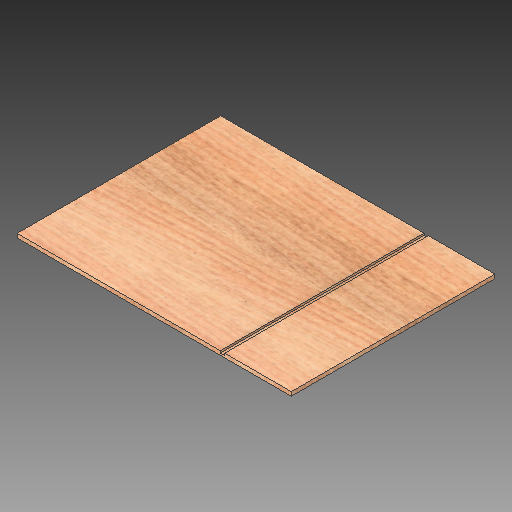
# Autodesk Inventor part: planche_bas
Saved by Autodesk Inventor 2019 (Build 230136000, 136)
## iProperties
Created: 2018-12-03
Part Number: planche_bas
Material: Wood (Birch)
Document SubType Name: Modeling
Designer: Bienvenue
Density: 0.55 g/cm^3
Appearance: Birch - Natural Polished
Author: Bienvenue
Autodesk Inventor part; units mm, degrees
ref_plane "YZ Plane" through (0, 0, 0) normal (1, 0, 0) x (0, 1, 0)
ref_plane "XZ Plane" through (0, 0, 0) normal (0, 1, 0) x (-1, 0, 0)
ref_plane "XY Plane" through (0, 0, 0) normal (0, 0, 1) x (1, 0, 0)
sketch "Sketch1" plane through (0, 0, 0) normal (0, 1, 0) x (-1, 0, 0)
  line L0 (0, 0) -> (412, 0)
  line L1 (412, 0) -> (412, -306)
  line L2 (412, -306) -> (0, -306)
  line L3 (0, -306) -> (0, 0)
  dimension "d0" = 306
  dimension "d1" = 412
  constraints: 8 end point, 2 parallel, 1 horizontal, 1 perpendicular
  measures "d0" distance of L2.end L0.start
  measures "d1" distance of L1.end L2.end
extrude "Extrusion1" add sketch "Sketch1" along normal blind 6
sketch "Sketch2" plane through (0, 6, 0) normal (0, 1, 0) x (1, 0, 0)
  line L0 (-412, 0) -> (0, 0) projected
  line L1 (0, 306) -> (-412, 306) projected
  line L2 (-106.5, 0) -> (-100, 0)
  line L3 (-100, 0) -> (-100, 306)
  line L4 (-100, 306) -> (-106.5, 306)
  line L5 (-106.5, 306) -> (-106.5, 0)
  line L6 (0, 0) -> (0, 306) projected
  dimension "d4" = 6.5
  dimension "d5" = 100
  constraints: 8 end point, 2 parallel, 2 point on line, 1 horizontal, 1 perpendicular
  measures "d4" distance between parallel lines of L3 L5
  measures "d5" distance between parallel lines of L6 L3
extrude "Extrusion2" cut sketch "Sketch2" against normal blind 3 contours L5 L1 L3 L0
body "Solid1"
